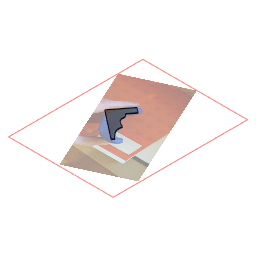
Jack Project Playdoh 1 v2 (Autodesk Fusion 360 design; units mm, degrees)
Autodesk Fusion 360 part; units mm, degrees
sketch "Sketch1" plane through (0, 0, 0) normal (0, 0, 1) x (1, 0, 0)
sketch "Sketch2" plane through (0, 0, 0) normal (0, 0, 1) x (1, 0, 0)
sketch "Sketch3" plane through (0, 0, 0) normal (0, 0, 1) x (1, 0, 0)
  spline S0 degree 5 poles (-14, 32) (-14.3895, 31.4851) (-15.1685, 30.4553) (-16.3369, 28.9105) (-17.8949, 26.8509) (-19.8423, 24.2763) (-21.4002, 22.2166) (-22.5687, 20.6719) (-23.3477, 19.6421) (-23.7371, 19.1271) knots 0 0 0 0 0 0 0.2 0.4 0.6 0.8 1 1 1 1 1 1
  spline S1 degree 5 poles (-23.7371, 19.1271) (-23.6286, 19.0196) (-23.4154, 18.8099) (-23.1068, 18.5109) (-22.7182, 18.144) (-22.2688, 17.7351) (-21.8503, 17.3674) (-21.4506, 17.0217) (-21.0527, 16.6685) (-20.6472, 16.2739) (-20.2432, 15.8058) (-19.8773, 15.2388) (-19.5934, 14.5553) (-19.4274, 13.7468) (-19.3866, 12.816) (-19.4408, 11.7765) (-19.5359, 10.6489) (-19.6029, 9.4577) (-19.568, 8.2277) (-19.3622, 6.9809) (-18.9321, 5.7329) (-18.2393, 4.4933) (-17.257, 3.2672) (-15.9683, 2.0559) (-14.3635, 0.8582) (-12.4382, -0.3286) (-10.6409, -1.2718) (-9.1487, -1.977) (-8.0898, -2.4463) (-7.5444, -2.6808) knots 0 0 0 0 0 0 0.04 0.08 0.12 0.16 0.2 0.24 0.28 0.32 0.36 0.4 0.44 0.48 0.52 0.56 0.6 0.64 0.68 0.72 0.76 0.8 0.84 0.88 0.92 0.96 1 1 1 1 1 1
  line L0 (-12.3379, -0.6203) -> (-2.7509, -4.7412)
  spline S2 degree 5 poles (-11.2333, -0.9391) (-11.0935, -0.9987) (-10.816, -1.1181) (-10.4065, -1.2971) (-9.874, -1.5357) (-9.2319, -1.8334) (-8.6159, -2.1302) (-8.0294, -2.4237) (-7.4796, -2.7126) (-6.9713, -2.9898) (-6.5274, -3.2606) (-6.188, -3.5438) (-5.9901, -3.8597) (-5.9578, -4.224) (-6.0817, -4.6362) (-6.3252, -5.0824) (-6.5795, -5.4514) (-6.7858, -5.727) (-6.9279, -5.9093) (-7, -6) knots 0 0 0 0 0 0 0.066667 0.133333 0.2 0.266667 0.333333 0.4 0.466667 0.533333 0.6 0.666667 0.733333 0.8 0.866667 0.933333 1 1 1 1 1 1
  line L1 (-6.329, -5.1562) -> (-7.671, -6.8438)
  line L2 (-8.3606, -2.2454) -> (-6.7282, -3.1161)
  spline S3 degree 5 poles (-7, -6) (-6.9977, -6.1998) (-6.994, -6.599) (-6.9916, -7.1969) (-6.9943, -7.9921) (-7.0038, -8.9848) (-7.0077, -9.9824) (-6.982, -10.9973) (-6.8862, -12.0505) (-6.6731, -13.1657) (-6.2989, -14.3631) (-5.7325, -15.6537) (-4.9685, -17.0317) (-4.0277, -18.4743) (-2.948, -19.9476) (-1.7784, -21.4117) (-0.5716, -22.8246) (0.6221, -24.148) (1.7619, -25.3512) (2.8226, -26.4164) (3.79, -27.3344) (4.4845, -27.9487) (4.9603, -28.342) (5.2575, -28.5743) (5.4011, -28.683) knots 0 0 0 0 0 0 0.05 0.1 0.15 0.2 0.25 0.3 0.35 0.4 0.45 0.5 0.55 0.6 0.65 0.7 0.75 0.8 0.85 0.9 0.95 1 1 1 1 1 1
  line L3 (-14, 32) -> (-23, 39)
  line L4 (-23, 39) -> (-48.0203, 6.831)
  line L5 (-48.0203, 6.831) -> (2.476, -32.4439)
  line L6 (5.4011, -28.683) -> (2.476, -32.4439)
  point P0 (-22, 17.5)
  point P1 (-20.6977, 16.3087)
  point P2 (-19.5, 14)
  point P3 (-19.5, 8)
  point P4 (-6, -4)
  point P5 (-7, -10)
  point P6 (-6, -15)
  point P7 (0.5, -24)
  constraint midpoint S1.end L0
  constraint coincident S1 S2.start
  constraint midpoint S2.end L1
  constraint midpoint S1.end L2
  constraint perpendicular L3 L4
  constraint perpendicular L4 L5
  constraint perpendicular L5 L6
extrude "Extrude1" add sketch "Sketch3" along normal blind 1 contours S0 S1 S2 S3 L3 L4 L5 L6
